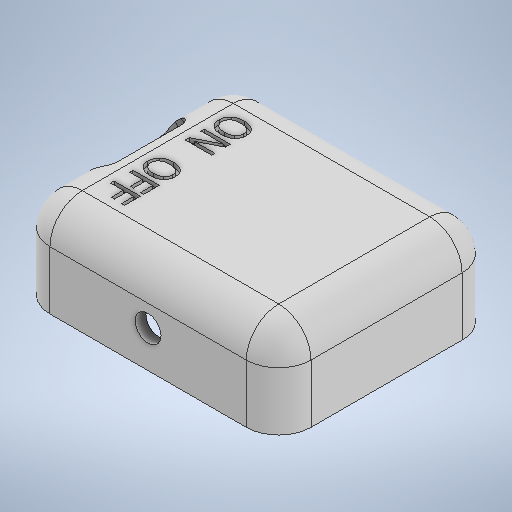
# Autodesk Inventor part: PCB_Deckel
Saved by Autodesk Inventor 2025.2 (Build 292293000, 293)
## iProperties
Created: 2024-11-12
Part Number: PCB_Deckel
Material: Generic
Document SubType Name: Modeling
Designer: matss
Density: 1 g/cm^3
Appearance: Default
Author: matss
Autodesk Inventor part; units mm, degrees
ref_plane "YZ Plane" through (0, 0, 0) normal (1, 0, 0) x (0, 1, 0)
ref_plane "XZ Plane" through (0, 0, 0) normal (0, 1, 0) x (-1, 0, 0)
ref_plane "XY Plane" through (0, 0, 0) normal (0, 0, 1) x (1, 0, 0)
sketch "Sketch1" plane through (0, 0, 0) normal (0, 1, 0) x (-1, 0, 0)
  line L0 (22.75, 22.5) -> (-22.75, 22.5)
  line L1 (-27.75, 17.5) -> (-27.75, -17.5)
  line L2 (-22.75, -22.5) -> (22.75, -22.5)
  line L3 (27.75, -17.5) -> (27.75, 17.5)
  arc A0 (27.75, 17.5) -> (22.75, 22.5) centre (22.75, 17.5) ccw
  arc A1 (22.75, -22.5) -> (27.75, -17.5) centre (22.75, -17.5) ccw
  arc A2 (-27.75, -17.5) -> (-22.75, -22.5) centre (-22.75, -17.5) ccw
  arc A3 (-22.75, 22.5) -> (-27.75, 17.5) centre (-22.75, 17.5) ccw
  line L4 (30.25, 17.5) -> (30.25, -17.5)
  arc A4 (22.75, -25) -> (30.25, -17.5) centre (22.75, -17.5) ccw
  line L5 (22.75, -25) -> (-22.75, -25)
  arc A5 (-30.25, -17.5) -> (-22.75, -25) centre (-22.75, -17.5) ccw
  line L6 (-30.25, -17.5) -> (-30.25, 17.5)
  arc A6 (-22.75, 25) -> (-30.25, 17.5) centre (-22.75, 17.5) ccw
  line L7 (-22.75, 25) -> (22.75, 25)
  arc A7 (30.25, 17.5) -> (22.75, 25) centre (22.75, 17.5) ccw
  point P0 (0, 0)
  point P1 (27.75, 22.5)
  point P2 (27.75, -22.5)
  point P3 (0, 22.5)
  point P4 (27.75, 0)
  dimension "d0" = 45
  dimension "d1" = 55.5
  dimension "d2" = 5
  dimension "d3" = 2.5
  constraints: 16 end point, 16 point on circle, 8 centre point, 8 tangent, 4 parallel, 4 point on line, 3 equal radius, 2 midpoint, 2 perpendicular, 1 horizontal, 1 horizontal alignment, 1 vertical alignment, 7 other
  measures "d0" distance of point (27.75, -22.5) point (27.75, 22.5)
  measures "d1" distance between parallel lines of L1 L3
  measures "d2" radius of A0
  measures "d3" distance between parallel lines of L3 L4
extrude "Extrusion1" add sketch "Sketch1" along normal blind 3 contours A0 L3 A1 L2 A2 L1 A3 L0 | L4 A4 L5 A5 L6 A6 L7 A7
extrude "Extrusion2" add sketch "Sketch1" against normal blind 18
fillet "Fillet1" radius 5 8 edges at (26.2855, 0, 21.0355) (0, 0, 22.5) (-26.2855, 0, 21.0355) (-27.75, 0, 0) (-26.2855, 0, -21.0355) (0, 0, -22.5) (26.2855, 0, -21.0355) (27.75, 0, 0)
fillet "Fillet2" radius 7.5 8 edges at (-28.0533, 3, -22.8033) (-30.25, 3, 0) (-28.0533, 3, 22.8033) (0, 3, 25) (28.0533, 3, 22.8033) (30.25, 3, 0) (28.0533, 3, -22.8033) (0, 3, -25)
sketch "Sketch2" plane through (22.75, -18, -25) normal (0, 0, -1) x (-1, 0, 0)
  arc A0 (53, 13.5) -> (45.5, 21) centre (45.5, 13.5) ccw construction
  line L0 (45.5, 13.5) -> (50.8033, 18.8033) construction
  line L1 (45.5, 13.5) -> (53, 13.5) construction
  point P0 (22.75, 18)
  dimension "d10" = 45
  constraints: 4 end point, 2 point on circle, 1 coincident
  measures "d10" angle of L1 L0
ref_plane "Work Plane1" through (-28.0533, 0.8033, -25) normal (-0.7071068, 0.7071068, 0) x (-0.7071068, -0.7071068, 0)
sketch "Sketch3" plane through (-28.0533, 0.8033, -25) normal (-0.7071068, 0.7071068, 0) x (-0.7071068, -0.7071068, 0)
  line L0 (-5.3033, 42.5) -> (-5.3033, 7.5) construction
  line L1 (5.3033, 7.5) -> (5.3033, 42.5) construction
  line L2 (-3.75, 15) -> (3.75, 15)
  line L3 (3.75, 15) -> (3.75, 35)
  line L4 (3.75, 35) -> (-3.75, 35)
  line L5 (-3.75, 35) -> (-3.75, 15)
  line L6 (-5.3033, 25) -> (5.3033, 25) construction
  point P0 (-19.2687, 25)
  point P1 (-3.75, 25)
  point P2 (0, 15)
  point P3 (0, 25)
  dimension "d11" = 7.5
  dimension "d12" = 20
  constraints: 10 end point, 5 midpoint, 2 parallel, 1 horizontal, 1 perpendicular, 1 point on line, 1 vertical alignment
  measures "d11" distance between parallel lines of L3 L5
  measures "d12" distance of L4.end L2.start
extrude "Extrusion3" cut sketch "Sketch3" against normal blind 10
fillet "Fillet3" radius 2.75 4 edges at (-23.3189, 1.3722, -10) (-23.3189, 1.3722, 10) (-28.8704, -3.6829, 10) (-28.8704, -3.6829, -10)
sketch "Sketch4" plane through (0, 3, 0) normal (0, 1, 0) x (1, 0, 0)
  line L0 (-22.75, -17.5) -> (-22.75, 17.5) projected
  line L1 (-14.75, 15.5) -> (-14.75, 4.589) construction
  line L2 (-14.75, 4.589) -> (-24.8324, 4.589) construction
  line L3 (-24.8324, 4.589) -> (-24.8324, 15.5) construction
  line L4 (-24.8324, 15.5) -> (-14.75, 15.5) construction
  line L5 (-14.75, -0.9745) -> (-14.75, -15.5) construction
  line L6 (-14.75, -15.5) -> (-17.8648, -15.5) construction
  line L7 (-17.8648, -15.5) -> (-17.8648, -0.9745) construction
  line L8 (-17.8648, -0.9745) -> (-14.75, -0.9745) construction
  line L9 (-22.75, 17.5) -> (22.75, 17.5) projected
  line L10 (22.75, -17.5) -> (-22.75, -17.5) projected
  spline S0 degree 2 poles (-15.575, 10.5698) (-15.9801, 10.224) (-17.1657, 9.8387) (-17.9264, 9.8387) knots 0 0 0 1 2 2 2
  spline S1 degree 2 poles (-17.9264, 9.8387) (-18.6674, 9.8387) (-19.8679, 10.2142) (-20.273, 10.5698) knots 0 0 0 1 2 2 2
  spline S2 degree 2 poles (-20.273, 10.5698) (-20.6978, 10.9453) (-21.1029, 11.9382) (-21.1029, 12.536) knots 0 0 0 1 2 2 2
  spline S3 degree 2 poles (-21.1029, 12.536) (-21.1029, 13.1535) (-20.683, 14.1415) (-20.273, 14.5021) knots 0 0 0 1 2 2 2
  spline S4 degree 2 poles (-20.273, 14.5021) (-19.8679, 14.8529) (-18.6773, 15.2283) (-17.9264, 15.2283) knots 0 0 0 1 2 2 2
  spline S5 degree 2 poles (-17.9264, 15.2283) (-17.1607, 15.2283) (-15.9949, 14.8479) (-15.575, 14.4972) knots 0 0 0 1 2 2 2
  spline S6 degree 2 poles (-15.575, 14.4972) (-15.1699, 14.1415) (-14.75, 13.1485) (-14.75, 12.536) knots 0 0 0 1 2 2 2
  spline S7 degree 2 poles (-14.75, 12.536) (-14.75, 11.9135) (-15.1847, 10.9156) (-15.575, 10.5698) knots 0 0 0 1 2 2 2
  spline S8 degree 2 poles (-17.9264, 10.6835) (-17.3238, 10.6835) (-16.3901, 10.9453) (-16.0838, 11.1824) knots 0 0 0 1 2 2 2
  spline S9 degree 2 poles (-16.0838, 11.1824) (-15.7676, 11.4245) (-15.4515, 12.1062) (-15.4515, 12.531) knots 0 0 0 1 2 2 2
  spline S10 degree 2 poles (-15.4515, 12.531) (-15.4515, 12.9707) (-15.7578, 13.6327) (-16.0838, 13.8846) knots 0 0 0 1 2 2 2
  spline S11 degree 2 poles (-16.0838, 13.8846) (-16.395, 14.1267) (-17.3336, 14.3836) (-17.9264, 14.3836) knots 0 0 0 1 2 2 2
  spline S12 degree 2 poles (-17.9264, 14.3836) (-19.1269, 14.3836) (-20.4014, 13.3758) (-20.4014, 12.531) knots 0 0 0 1 2 2 2
  spline S13 degree 2 poles (-20.4014, 12.531) (-20.4014, 11.6863) (-19.1269, 10.6835) (-17.9264, 10.6835) knots 0 0 0 1 2 2 2
  line L11 (-20.9744, 4.5875) -> (-20.9744, 5.4964)
  line L12 (-20.9744, 5.4964) -> (-15.7182, 8.1937)
  line L13 (-15.7182, 8.1937) -> (-20.9744, 8.1937)
  line L14 (-20.9744, 8.1937) -> (-20.9744, 8.9495)
  line L15 (-20.9744, 8.9495) -> (-14.8784, 8.9495)
  line L16 (-14.8784, 8.9495) -> (-14.8784, 7.7985)
  line L17 (-14.8784, 7.7985) -> (-19.7049, 5.3433)
  line L18 (-19.7049, 5.3433) -> (-14.8784, 5.3433)
  line L19 (-14.8784, 5.3433) -> (-14.8784, 4.5875)
  line L20 (-14.8784, 4.5875) -> (-20.9744, 4.5875)
  spline S14 degree 2 poles (-15.575, -5.9046) (-15.9801, -6.2504) (-17.1657, -6.6357) (-17.9264, -6.6357) knots 0 0 0 1 2 2 2
  spline S15 degree 2 poles (-17.9264, -6.6357) (-18.6674, -6.6357) (-19.8679, -6.2603) (-20.273, -5.9046) knots 0 0 0 1 2 2 2
  spline S16 degree 2 poles (-20.273, -5.9046) (-20.6978, -5.5292) (-21.1029, -4.5362) (-21.1029, -3.9385) knots 0 0 0 1 2 2 2
  spline S17 degree 2 poles (-21.1029, -3.9385) (-21.1029, -3.321) (-20.683, -2.333) (-20.273, -1.9724) knots 0 0 0 1 2 2 2
  spline S18 degree 2 poles (-20.273, -1.9724) (-19.8679, -1.6216) (-18.6773, -1.2462) (-17.9264, -1.2462) knots 0 0 0 1 2 2 2
  spline S19 degree 2 poles (-17.9264, -1.2462) (-17.1607, -1.2462) (-15.9949, -1.6266) (-15.575, -1.9773) knots 0 0 0 1 2 2 2
  spline S20 degree 2 poles (-15.575, -1.9773) (-15.1699, -2.333) (-14.75, -3.3259) (-14.75, -3.9385) knots 0 0 0 1 2 2 2
  spline S21 degree 2 poles (-14.75, -3.9385) (-14.75, -4.5609) (-15.1847, -5.5588) (-15.575, -5.9046) knots 0 0 0 1 2 2 2
  spline S22 degree 2 poles (-17.9264, -5.791) (-17.3238, -5.791) (-16.3901, -5.5292) (-16.0838, -5.2921) knots 0 0 0 1 2 2 2
  spline S23 degree 2 poles (-16.0838, -5.2921) (-15.7676, -5.05) (-15.4515, -4.3683) (-15.4515, -3.9434) knots 0 0 0 1 2 2 2
  spline S24 degree 2 poles (-15.4515, -3.9434) (-15.4515, -3.5038) (-15.7578, -2.8418) (-16.0838, -2.5899) knots 0 0 0 1 2 2 2
  spline S25 degree 2 poles (-16.0838, -2.5899) (-16.395, -2.3478) (-17.3336, -2.0909) (-17.9264, -2.0909) knots 0 0 0 1 2 2 2
  spline S26 degree 2 poles (-17.9264, -2.0909) (-19.1269, -2.0909) (-20.4014, -3.0987) (-20.4014, -3.9434) knots 0 0 0 1 2 2 2
  spline S27 degree 2 poles (-20.4014, -3.9434) (-20.4014, -4.7882) (-19.1269, -5.791) (-17.9264, -5.791) knots 0 0 0 1 2 2 2
  line L21 (-15.5997, -11.1707) -> (-15.5997, -8.3351)
  line L22 (-15.5997, -8.3351) -> (-17.3188, -8.3351)
  line L23 (-17.3188, -8.3351) -> (-17.3188, -11.0521)
  line L24 (-17.3188, -11.0521) -> (-18.0401, -11.0521)
  line L25 (-18.0401, -11.0521) -> (-18.0401, -8.3351)
  line L26 (-18.0401, -8.3351) -> (-20.9744, -8.3351)
  line L27 (-20.9744, -8.3351) -> (-20.9744, -7.525)
  line L28 (-20.9744, -7.525) -> (-14.8784, -7.525)
  line L29 (-14.8784, -7.525) -> (-14.8784, -11.1707)
  line L30 (-14.8784, -11.1707) -> (-15.5997, -11.1707)
  line L31 (-15.5997, -15.5426) -> (-15.5997, -12.707)
  line L32 (-15.5997, -12.707) -> (-17.3188, -12.707)
  line L33 (-17.3188, -12.707) -> (-17.3188, -15.4241)
  line L34 (-17.3188, -15.4241) -> (-18.0401, -15.4241)
  line L35 (-18.0401, -15.4241) -> (-18.0401, -12.707)
  line L36 (-18.0401, -12.707) -> (-20.9744, -12.707)
  line L37 (-20.9744, -12.707) -> (-20.9744, -11.8969)
  line L38 (-20.9744, -11.8969) -> (-14.8784, -11.8969)
  line L39 (-14.8784, -11.8969) -> (-14.8784, -15.5426)
  line L40 (-14.8784, -15.5426) -> (-15.5997, -15.5426)
  point P0 (0, 0)
  point P1 (-24.6911, 7.25)
  point P2 (-27.2988, 10)
  point P3 (-27.2988, -10)
  dimension "d16" = 2
  dimension "d17" = 2
  dimension "d18" = 8
  constraints: 1 vertical alignment, 4 other
  measures "d16" distance from line of L9 L1.start
  measures "d17" distance from line of L10 L5.end
  measures "d18" distance from line of L0 L1.start
emboss "Emboss1" sketch "Sketch4" operation cut depth 1 direction (0, -1, 0)
ref_plane "Arbeitsebene2" through (-30.25, -18, 17.5) normal (0, 0, -1) x (0, 1, 0)
sketch "Skizze5" plane through (-30.25, -18, 17.5) normal (0, 0, -1) x (0, 1, 0)
  line L0 (13, 2.5) -> (0, 2.5) projected
  line L1 (0, 7.5) -> (0, 0) projected
  circle A0 centre (2.5, 2.5) radius 1
  line L2 (13, 58) -> (0, 58) projected
  line L3 (13, 2.5) -> (0, 58) construction
  line L4 (13, 58) -> (0, 2.5) construction
  line L5 (6.5, 30.25) -> (9.2319, 30.25) construction
  circle A1 centre (2.5, 58) radius 1
  point P0 (18, 30.25)
  point P1 (1.5, 58)
  point P2 (3.5, 58)
  point P3 (1.5, 2.5)
  point P4 (3.5, 2.5)
  dimension "d21" = 2.5
  dimension "d22" = 2
  constraints: 6 end point, 2 centre point, 1 coincident, 1 horizontal, 1 midpoint, 1 point on line, 1 symmetric about line, 1 other
  measures "d21" distance from line of L1 point (2.5, 2.5)
  measures "d22" diameter of A0
extrude "Extrusion4" add sketch "Skizze5" along normal blind 38 and the other way blind 3 contours L0 A0 | A1 L2 picked at (2.6894, 2.7743) picked at (2.6182, 57.6883)
sketch "Skizze6" plane through (22.75, -18, -25) normal (0, 0, -1) x (-1, 0, 0)
  line L0 (7.005, 12.6) -> (15.005, 12.6)
  line L1 (15.005, 12.6) -> (15.005, 9.1)
  line L2 (15.005, 9.1) -> (7.005, 9.1)
  line L3 (7.005, 9.1) -> (7.005, 12.6)
  line L4 (45.5, 0) -> (0, 0) projected
  line L5 (7.005, 12.6) -> (15.005, 9.1) construction
  line L6 (7.005, 9.1) -> (15.005, 12.6) construction
  line L7 (5.505, 7.35) -> (16.505, 7.35)
  line L8 (17.505, 8.35) -> (17.505, 13.35)
  line L9 (16.505, 14.35) -> (5.505, 14.35)
  line L10 (4.505, 13.35) -> (4.505, 8.35)
  line L11 (4.505, 7.35) -> (17.505, 14.35) construction
  line L12 (17.505, 7.35) -> (4.505, 14.35) construction
  arc A0 (5.505, 14.35) -> (4.505, 13.35) centre (5.505, 13.35) ccw
  arc A1 (4.505, 8.35) -> (5.505, 7.35) centre (5.505, 8.35) ccw
  arc A2 (16.505, 7.35) -> (17.505, 8.35) centre (16.505, 8.35) ccw
  arc A3 (17.505, 13.35) -> (16.505, 14.35) centre (16.505, 13.35) ccw
  point P0 (22.75, 18)
  point P1 (11.005, 10.85)
  dimension "d27" = 9.1
  dimension "d28" = 3.5
  dimension "d29" = 7.005
  dimension "d30" = 8
  dimension "d31" = 13
  dimension "d33" = 7
  dimension "d34" = 1
  constraints: 24 end point, 8 point on circle, 8 point on line, 8 tangent, 4 centre point, 4 parallel, 3 equal radius, 3 midpoint, 2 horizontal, 2 perpendicular
  measures "d27" distance between parallel lines of L4 L2
  measures "d28" distance of L0.end L1.end
  measures "d29" distance from line of L4.end L3
  measures "d30" distance between parallel lines of L1 L3
  measures "d31" distance of L11.start L12.start
  measures "d33" distance of L12.start L11.end
  measures "d34" radius of A0
extrude "Extrusion5" cut sketch "Skizze6" against normal blind 3 contours L0 L1 L2 L3 | A1 L10 A0 L9 A3 L8 A2 L7
sketch "Sketch7" plane through (22.75, -18, -25) normal (0, 0, -1) x (-1, 0, 0)
  line L0 (17.505, 13.35) -> (17.505, 8.35) construction
  circle A0 centre (37.505, 10.85) radius 2
  point P0 (22.75, 18)
  point P1 (17.505, 10.85)
  point P2 (17.505, 10.85)
  dimension "d37" = 4
  dimension "d38" = 20
  constraints: 2 midpoint, 1 centre point, 1 horizontal alignment
  measures "d37" diameter of A0
  measures "d38" distance of point (17.505, 10.85) A0.centre
extrude "Extrusion6" cut sketch "Sketch7" against normal blind 10
sketch "Sketch8" plane through (0, 0, 0) normal (0, -1, 0) x (1, 0, 0)
  circle A0 centre (-9, 0) radius 2.5
  circle A1 centre (-9, 0) radius 3.5
  point P0 (0, 0)
  dimension "d41" = 5
  dimension "d42" = 7
  dimension "d43" = 9
  constraints: 2 centre point, 1 coincident, 1 horizontal alignment
  measures "d41" diameter of A0
  measures "d42" diameter of A1
  measures "d43" distance of point (0, 0) A0.centre
extrude "Extrusion7" add sketch "Sketch8" along normal blind 6
sketch "Sketch9" plane through (-9, 0, 0) normal (0, -1, 0) x (1, 0, 0)
  circle A0 centre (0, 0) radius 2.5 projected
  point P0 (9, 0)
extrude "Extrusion8" cut sketch "Sketch9" against normal blind 1.75
chamfer "Chamfer1" distance 2 angle 45 1 edges at (-12.5, 0, 0)
sketch "Sketch10" plane through (-22.75, -18, 25) normal (0, 0, 1) x (1, 0, 0)
  circle A0 centre (22.75, 8.5) radius 3
  line L0 (0, 13.5) -> (45.5, 13.5) projected
  line L1 (0, 0) -> (0, 13.5) projected
  point P0 (22.75, 18)
  point P1 (22.75, 13.5)
  point P2 (0, 6.75)
  point P3 (22.75, 13.5)
  point P4 (22.75, 13.5)
  dimension "d51" = 6
  dimension "d60" = 5
  constraints: 4 midpoint, 1 centre point, 1 vertical alignment
  measures "d51" diameter of A0
  measures "d60" distance of point (22.75, 13.5) A0.centre
extrude "Extrusion9" cut sketch "Sketch10" against normal blind 3
body "Solid1"
